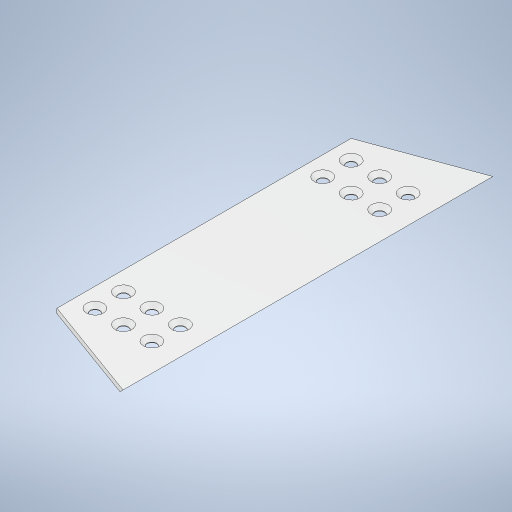
# Autodesk Inventor part: Wedge
Saved by Autodesk Inventor 2023.2 (Build 272271000, 271)
## iProperties
Created: 2024-03-02
Part Number: Wedge
Material: Aluminum 6061
Document SubType Name: Modeling
Designer: Nathan Cai
Mass: 24.0653 g
Surface Area: 121.334 cm^2
Volume: 8.91306 cm^3
Density: 2.7 g/cm^3
Appearance: Aluminum - Flat
Author: Nathan Cai
Autodesk Inventor part; units mm, degrees
ref_plane "YZ Plane" through (0, 0, 0) normal (1, 0, 0) x (0, 1, 0)
ref_plane "XZ Plane" through (0, 0, 0) normal (0, 1, 0) x (-1, 0, 0)
sketch "Sketch1" plane through (0, 0, 0) normal (0, 1, 0) x (-1, 0, 0)
  line L0 (-19.05, 49.2125) -> (19.05, 49.2125)
  line L1 (19.05, 49.2125) -> (19.05, -49.2125)
  line L2 (19.05, -49.2125) -> (-19.05, -49.2125)
  line L3 (-19.05, -49.2125) -> (-19.05, 49.2125)
  line L4 (-19.05, 49.2125) -> (19.05, -49.2125) construction
  line L5 (19.05, 49.2125) -> (-19.05, -49.2125) construction
  line L6 (19.05, 0) -> (-19.05, 0) construction
  line L7 (-19.05, -49.2125) -> (19.05, -49.2125) construction
  line L8 (19.05, -49.2125) -> (19.05, -87.3125)
  line L9 (19.05, -87.3125) -> (-19.05, -87.3125)
  line L10 (-19.05, -87.3125) -> (-19.05, -49.2125)
  line L11 (19.05, -49.2125) -> (-19.05, -63.0798)
  line L12 (19.05, 49.2125) -> (-19.05, 49.2125) construction
  line L13 (-19.05, 49.2125) -> (19.05, 49.2125) construction
  line L14 (19.05, 49.2125) -> (19.05, 87.3125)
  line L15 (19.05, 87.3125) -> (-19.05, 87.3125)
  line L16 (-19.05, 87.3125) -> (-19.05, 49.2125)
  line L17 (19.05, 49.2125) -> (-19.05, 63.0798)
  line L18 (19.05, 42.8625) -> (-19.05, 42.8625) construction
  line L19 (-19.05, -63.0798) -> (9.525, -87.3125)
  line L20 (-19.05, 63.0798) -> (9.525, 87.3125)
  point P0 (0, 0)
  point P1 (12.7, 42.8625)
  point P2 (3.175, 42.8625)
  point P3 (-6.35, 42.8625)
  point P4 (12.7, 33.3375)
  point P5 (3.175, 33.3375)
  point P6 (-6.35, 33.3375)
  point P7 (12.7, -42.8625)
  point P8 (3.175, -42.8625)
  point P9 (-6.35, -42.8625)
  point P10 (12.7, -33.3375)
  point P11 (3.175, -33.3375)
  point P12 (-6.35, -33.3375)
  point P13 (19.05, 49.2125)
  point P14 (9.525, 87.3125)
  point P15 (19.05, 49.2125)
  point P16 (-19.05, 63.0798)
  dimension "d0" = 38.1
  dimension "d1" = 98.425
  dimension "d2" = 38.1
  dimension "d3" = 38.1
  dimension "d5" = 20
  dimension "d20" = 6.35
  dimension "d23" = 9.525
  dimension "d26" = 9.525
  dimension "d29" = 6.35
  dimension "d33" = 28.575
  constraints: 42 end point, 13 symmetric about line, 6 point on line, 4 midpoint, 4 parallel, 3 horizontal, 3 perpendicular, 1 vertical, 5 other
  measures "d0" distance of L1.end L2.end
  measures "d1" distance of L0.end L1.end
  measures "d2" distance of L8.end L9.end
  measures "d3" distance of L7.end L8.end
  measures "d5" angle of L2 L11
  measures "d20" distance from line of L1 point (12.7, 42.863)
  measures "d23" distance of point (12.7, 42.863) point (3.175, 42.863)
  measures "d26" distance of point (12.7, 42.863) point (12.7, 33.338)
  measures "d29" distance between parallel lines of L0 L18
  measures "d33" distance from line of L10 L19.end
extrude "Extrusion1" add sketch "Sketch1" against normal blind 1.5875 contours L16 L17 L0 | L0 L1 L2 L3 | L2 L11 L10
ref_plane "Work Plane2" through (19.05, -1.5, 88.9) normal (-0.7071, -0.7071, 0) x (0, 0, 1)
feature "Bend Part3" [suppressed]
feature "Bend Part4" [suppressed]
sketch "Sketch2" plane through (19.05, -1.5, 88.9) normal (-0.7071, -0.7071, 0) x (0, 0, 1)
  line L0 (-10.6966, 1.0607) -> (-167.1034, 1.0607)
  line L1 (-167.1034, 1.0607) -> (-167.1034, -24.3393)
  line L2 (-167.1034, -24.3393) -> (-10.6966, -24.3393)
  line L3 (-10.6966, -24.3393) -> (-10.6966, 1.0607)
  line L4 (-10.6966, 1.0607) -> (-167.1034, 1.0607)
  line L5 (-167.1034, 1.0607) -> (-167.1034, 3.4419)
  line L6 (-167.1034, 3.4419) -> (-10.6966, 3.4419)
  line L7 (-10.6966, 3.4419) -> (-10.6966, 1.0607)
  point P0 (-88.9, 14.531)
  point P1 (-153.5673, 1.0607)
  point P2 (-167.1034, -7.4895)
  point P3 (-10.6966, -7.4895)
  dimension "d31" = 25.4
  dimension "d32" = 2.3813
  constraints: 16 end point, 4 parallel, 4 point on line, 2 horizontal, 2 perpendicular
  measures "d31" distance between parallel lines of L0 L2
  measures "d32" distance of L4.end L5.end
extrude "Extrusion2" cut sketch "Sketch2" along normal through all both and the other way through all
hole "Hole1" at (-12.7, 0, 42.8625) at (-3.175, 0, 42.8625) at (6.35, 0, 42.8625) at (-12.7, 0, 33.3375) at (-3.175, 0, 33.3375) at (6.35, 0, 33.3375) at (6.35, 0, -33.3375) at (-3.175, 0, -33.3375) at (-12.7, 0, -33.3375) at (6.35, 0, -42.8625) at (-3.175, 0, -42.8625) at (-12.7, 0, -42.8625) direction (0, -1, 0) diameter 3.2766 end through all countersink diameter 5.715 countersink angle 82 clearance for "Flat Head Machine Screw (82)" size "#4" standard "Ansi Unified Screw Threads"
equation "\"d0\" = d2"
body "Solid1"
